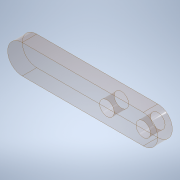
# Autodesk Inventor part: カウンター先端
Saved by Autodesk Inventor 2020.2 (Build 242310000, 310)
## iProperties
Created: 2020-04-05
Part Number: カウンター先端
Material: ポリカーボネート、スモーク
Document SubType Name: Modeling
Designer: aoyama
Density: 1.2 g/cm^3
Appearance: ポリカーボネート - スモーク
Mass: 0.590894 g
Surface Area: 5.91372 cm^2
Volume: 0.492412 cm^3
Author: aoyama
Autodesk Inventor part; units mm, degrees
ref_plane "YZ Plane" through (0, 0, 0) normal (1, 0, 0) x (0, 1, 0)
ref_plane "XZ Plane" through (0, 0, 0) normal (0, 1, 0) x (-1, 0, 0)
ref_plane "XY Plane" through (0, 0, 0) normal (0, 0, 1) x (1, 0, 0)
sketch "スケッチ1" plane through (0, 0, 0) normal (0, 0, 1) x (1, 0, 0)
  line L0 (0, 0) -> (-7.5, 0) construction
  line L1 (0, 3) -> (-7.5, 3)
  line L2 (-7.5, -3) -> (0, -3)
  arc A0 (0, -3) -> (0, 3) centre (0, 0) ccw
  arc A1 (-7.5, 3) -> (-7.5, -3) centre (-7.5, 0) ccw
  circle A2 centre (-7.5, 0) radius 1.5
  circle A3 centre (0, 0) radius 1.5
  line L3 (0, 0) -> (-25, 0) construction
  line L4 (0, -3) -> (-25, -3)
  line L5 (-25, 3) -> (0, 3)
  arc A4 (0, -3) -> (0, 3) centre (0, 0) ccw
  arc A5 (-25, 3) -> (-25, -3) centre (-25, 0) ccw
  circle A6 centre (-25, 0) radius 1.5
  point P0 (-3.75, 0)
  point P1 (-12.5, 0)
  dimension "d0" = 6
  dimension "d1" = 7.5
  dimension "d2" = 3
  dimension "d3" = 3
  dimension "d4" = 25
  dimension "d7" = 3
  constraints: 16 end point, 8 point on circle, 8 tangent, 7 centre point, 3 coincident, 2 midpoint, 2 parallel
  measures "d0" diameter of A1
  measures "d1" distance of L0.start L0.end
  measures "d2" diameter of A2
  measures "d3" diameter of A3
  measures "d4" distance of L3.end L0.start
  measures "d7" diameter of A6
extrude "押し出し1" add sketch "スケッチ1" along normal blind 3 contours A0 L2 A1 L1 | A1 L4 A5 L5 | A6
